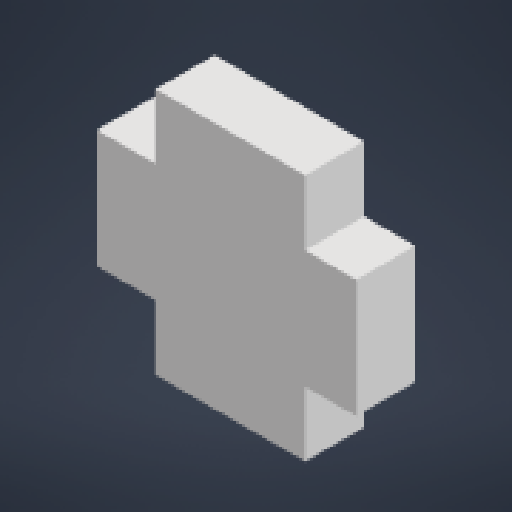
# Autodesk Inventor part: Part7
Saved by Autodesk Inventor 2026.2 (Build 302298000, 298)
## iProperties
Created: 2026-04-17
Part Number: Part7
Material: Generic
Document SubType Name: Modeling
Designer: danda
Density: 1 g/cm^3
Appearance: Default
Author: danda
Autodesk Inventor part; units mm, degrees
ref_plane "YZ Plane" through (0, 0, 0) normal (1, 0, 0) x (0, 1, 0)
ref_plane "XZ Plane" through (0, 0, 0) normal (0, 1, 0) x (-1, 0, 0)
ref_plane "XY Plane" through (0, 0, 0) normal (0, 0, 1) x (1, 0, 0)
sketch "Sketch1" plane through (0, 0, 0) normal (0, 0, 1) x (1, 0, 0)
  line L0 (9.2486, 28.2975) -> (31.2486, 28.2975)
  line L1 (31.2486, 28.2975) -> (31.2486, 7.2975)
  line L2 (31.2486, 7.2975) -> (9.2486, 7.2975)
  line L3 (9.2486, 7.2975) -> (9.2486, 28.2975)
  line L4 (14.2486, 17.9108) -> (26.9185, 17.9108)
  line L5 (26.9185, 28.2975) -> (26.9185, 7.2975)
  line L6 (26.9185, 11.9108) -> (14.2486, 11.9108)
  line L7 (14.2486, 7.2975) -> (14.2486, 28.2975)
  line L8 (31.2486, 25.2975) -> (31.2486, 10.2975)
  line L9 (31.2486, 25.2975) -> (26.9185, 22.7975)
  line L10 (31.2486, 25.2975) -> (36.2486, 25.2975) construction
  line L11 (31.2486, 10.2975) -> (26.9185, 12.7975)
  line L12 (31.2486, 10.2975) -> (36.2486, 10.2975) construction
  line L13 (20.2486, 30.1411) -> (20.2486, -2.0626)
  line L14 (9.2486, 25.2975) -> (13.5787, 22.7975)
  line L15 (9.2486, 10.2975) -> (13.5787, 12.7975)
  line L16 (13.5787, 22.7975) -> (9.2486, 22.7975)
  line L17 (13.5787, 22.7975) -> (14.2486, 22.7975)
  line L18 (14.2486, 12.7975) -> (9.2486, 12.7975)
  line L19 (26.9185, 22.7975) -> (31.9185, 22.7975)
  line L20 (31.9185, 22.7975) -> (31.9185, 7.2975)
  line L21 (31.9185, 7.2975) -> (31.2486, 7.2975)
  line L22 (26.9185, 12.7975) -> (31.9185, 12.7975)
  line L23 (31.9185, 22.7975) -> (31.9185, 28.2975)
  line L24 (31.9185, 28.2975) -> (31.2486, 28.2975)
  point P0 (0, 0)
  point P1 (14.2486, 22.024)
  point P2 (9.2486, 25.2975)
  point P3 (9.2486, 10.2975)
  point P4 (14.2486, 12.7975)
  point P5 (31.2486, 12.7975)
  point P6 (31.2486, 22.7975)
  dimension "d0" = 22
  dimension "d1" = 21
  dimension "d2" = 5
  dimension "d3" = 15
  dimension "d4" = 3
  dimension "d5" = 150
  dimension "d6" = 150
  dimension "d7" = 11
  dimension "d10" = 10
  dimension "d11" = 5
  constraints: 50 end point, 19 point on line, 9 perpendicular, 4 parallel, 4 symmetric about line, 3 horizontal, 2 equal length, 1 vertical
  measures "d0" distance of L1.end L2.end
  measures "d1" distance of L0.end L1.end
  measures "d2" distance between parallel lines of L3 L7
  measures "d3" distance of L8.start L8.end
  measures "d4" distance of L0.end L8.start
  measures "d5" angle of L9 L10
  measures "d6" angle of L12 L11
  measures "d7" distance between parallel lines of L3 L13
  measures "d10" distance of L15.end L14.end
  measures "d11" distance of L9.end L19.end
extrude "Extrusion1" add sketch "Sketch1" along normal blind 5 contours L0 L13 L4 L7 | L0 L5 L4 L13 | L7 L18 L3 L16 L17 | L13 L6 L7 L4 | L4 L5 L6 L13 | L19 L1 L22 L5 | L13 L2 L7 L6 | L6 L5 L2 L13
body "Solid1"
